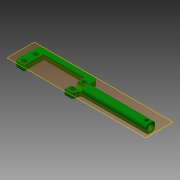
# Autodesk Inventor part: Fork2
Saved by Autodesk Inventor 2014 SP1 (Build 180222100, 222)
## iProperties
Created: 2017-01-17
Part Number: Fork2
Material: Generic
Document SubType Name: Modeling
Designer: danielsikar
Density: 1 g/cm^3
Appearance: Dark Green
Author: danielsikar
Autodesk Inventor part; units mm, degrees
ref_plane "YZ Plane" through (0, 0, 0) normal (1, 0, 0) x (0, 1, 0)
ref_plane "XZ Plane" through (0, 0, 0) normal (0, 1, 0) x (-1, 0, 0)
sketch "Sketch1" plane through (0, 0, 0) normal (0, 0, 1) x (1, 0, 0)
  line L0 (0, 0) -> (6.8, 0)
  line L1 (6.8, 0) -> (6.8, -20)
  line L2 (6.8, -20) -> (0, -20)
  line L3 (0, -20) -> (0, 0)
  arc A0 (5.8439, -3.1) -> (5.8439, -5.5) centre (4, -4.3) ccw projected
  line L4 (5.8439, -3.1) -> (6.8, -3.1) projected
  line L5 (6.8, -5.5) -> (5.8439, -5.5) projected
  arc A1 (5.8439, -14.5) -> (5.8439, -16.9) centre (4, -15.7) ccw projected
  line L6 (5.8439, -14.5) -> (6.8, -14.5) projected
  line L7 (6.8, -16.9) -> (5.8439, -16.9) projected
  dimension "d0" = 6.8
  dimension "d1" = 20
  constraints: 8 end point, 2 parallel, 1 horizontal, 1 perpendicular, 1 other
  measures "d0" distance of L1.end L2.end
  measures "d1" distance of L0.end L1.end
extrude "Extrusion1" add sketch "Sketch1" along normal blind 5
sketch "Sketch2" plane through (0, 0, 0) normal (0, 0, -1) x (-1, 0, 0)
  line L0 (-6.8, 0) -> (-6.8, -20) projected
  arc A0 (-5.8439, -5.5) -> (-5.8439, -3.1) centre (-4, -4.3) ccw projected
  line L1 (-5.8439, -5.5) -> (-6.8, -5.5) projected
  line L2 (-6.8, -3.1) -> (-5.8439, -3.1) projected
  arc A1 (-5.8439, -16.9) -> (-5.8439, -14.5) centre (-4, -15.7) ccw projected
  line L3 (-5.8439, -16.9) -> (-6.8, -16.9) projected
  line L4 (-6.8, -14.5) -> (-5.8439, -14.5) projected
extrude "Extrusion2" cut sketch "Sketch2" against normal blind 5
ref_plane "Work Plane1" through (-20.15, -14.5, 0) normal (1, 0, 0) x (0, 0, -1)
mirror "Mirror1" about plane through (-20.15, -14.5, 0) normal (1, 0, 0) of "Extrusion2", "Extrusion1"
sketch "Sketch3" plane through (0, 0, 0) normal (0, 1, 0) x (1, 0, 0)
  line L0 (6.8, -5) -> (-47.1, -5)
  line L1 (-47.1, -5) -> (-47.1, 0)
  line L2 (-47.1, 0) -> (6.8, 0)
  line L3 (6.8, 0) -> (6.8, -5)
  dimension "d7" = 53.9
  constraints: 8 end point, 2 parallel, 1 horizontal, 1 perpendicular
  measures "d7" distance of L1.end L2.end
extrude "Extrusion3" add sketch "Sketch3" along normal blind 5
sketch "Sketch5" plane through (6.8, -14.5, 0) normal (1, 0, 0) x (0, 0, -1)
  line L0 (0, 9) -> (-5, 9) projected
  line L1 (-5, 0) -> (-5, 9) projected
  line L2 (-5, 0) -> (0, 0) projected
  line L3 (0, 9) -> (0, 0) projected
  point P0 (0, 14.5)
extrude "Extrusion5" add sketch "Sketch5" along normal blind 70
sketch "Sketch6" plane through (0, 0, 5) normal (0, 0, 1) x (1, 0, 0)
  line L0 (5.8439, -14.5) -> (76.8, -14.5) projected
  line L1 (76.8, -5.5) -> (76.8, -14.5) projected
  line L2 (76.8, -5.5) -> (11.825, -5.5)
  line L3 (11.825, -5.5) -> (11.825, -14.5)
  line L4 (11.825, -14.5) -> (76.8, -14.5)
  line L5 (76.8, -14.5) -> (76.8, -5.5)
  constraints: 8 end point, 2 parallel, 1 horizontal, 1 perpendicular, 1 point on line
extrude "Extrusion6" add sketch "Sketch6" along normal blind 4
sketch "Sketch7" plane through (6.8, -3.1, 5) normal (1, 0, 0) x (0, 0, -1)
  line L0 (0, 8.1) -> (5, 8.1)
  line L1 (5, 8.1) -> (5, -16.9)
  line L2 (5, -16.9) -> (0, -16.9)
  line L3 (0, -16.9) -> (0, 8.1)
  point P0 (5, 3.1)
  dimension "d16" = 25
  constraints: 8 end point, 2 parallel, 1 horizontal, 1 perpendicular
  measures "d16" distance between parallel lines of L2 L0
extrude "Extrusion7" add sketch "Sketch7" along normal blind 2
sketch "Sketch9" plane through (0, 0, 9) normal (0, 0, 1) x (1, 0, 0)
  line L0 (76.8, -14.5) -> (76.8, -5.5) projected
  circle A0 centre (72.8, -10) radius 1.7
  point P0 (0, 0)
  dimension "d21" = 3.4
  dimension "d22" = 4
  constraints: 1 centre point
  measures "d21" diameter of A0
  measures "d22" distance from line of L0 A0.centre
extrude "Extrusion8" cut sketch "Sketch9" against normal through all
sketch "Sketch10" plane through (76.8, -14.5, 0) normal (1, 0, 0) x (0, 0, -1)
  circle A0 centre (-4.5, 4.5) radius 3
  point P0 (0, 14.5)
  dimension "d25" = 6
  constraints: 1 centre point
  measures "d25" diameter of A0
extrude "Extrusion9" cut sketch "Sketch10" against normal blind 80
fillet "Fillet1" radius 3 4 edges at (44.3125, -14.5, 9) (44.3125, -5.5, 9) (42.8, -5.5, 0) (42.8, -14.5, 0)
fillet "Fillet2" radius 3 4 edges at (8.8, -5.5, 4) (8.8, -6.3787, 0.8787) (8.8, -14.5, 4) (8.8, -13.6213, 0.8787)
fillet "Fillet3" radius 3 2 edges at (8.8, 5, 2.5) (8.8, -20, 2.5)
sketch "Sketch12" plane through (0, -20, 0) normal (-1, 0, 0) x (0, 0, 1)
  arc A0 (5, 12.958) -> (5, 7.042) centre (4.5, 10) ccw projected
  line L0 (5, 20) -> (5, 12.958) projected
  line L1 (0, 20) -> (5, 20) projected
  line L2 (0, 0) -> (0, 20) projected
  line L3 (0, 0) -> (5, 0) projected
  line L4 (5, 7.042) -> (5, 0) projected
extrude "Extrusion10" cut sketch "Sketch12" against normal blind 0.25
sketch "Sketch13" plane through (-40.3, -20, 5) normal (1, 0, 0) x (0, 0, -1)
  line L0 (5, 0) -> (5, 20) projected
  line L1 (5, 20) -> (0, 20) projected
  line L2 (0, 20) -> (0, 0) projected
  line L3 (5, 0) -> (0, 0) projected
extrude "Extrusion11" cut sketch "Sketch13" against normal blind 0.25
sketch "Sketch14" plane through (-47.1, -3.1, 0) normal (-1, 0, 0) x (0, 0, 1)
  line L0 (0, 8.1) -> (5, 8.1)
  line L1 (5, 8.1) -> (5, -16.9)
  line L2 (5, -16.9) -> (0, -16.9)
  line L3 (0, -16.9) -> (0, 8.1)
  point P0 (0, 3.1)
  dimension "d35" = 25
  constraints: 8 end point, 2 parallel, 1 horizontal, 1 perpendicular
  measures "d35" distance between parallel lines of L2 L0
extrude "Extrusion12" add sketch "Sketch14" along normal blind 3
fillet "Fillet4" radius 3 2 edges at (-50.1, 5, 2.5) (-50.1, -20, 2.5)
ref_plane "ConstraintPlane" through (0, 0, 4.5) normal (0, 0, 1) x (1, 0, 0)
body "Solid1"
